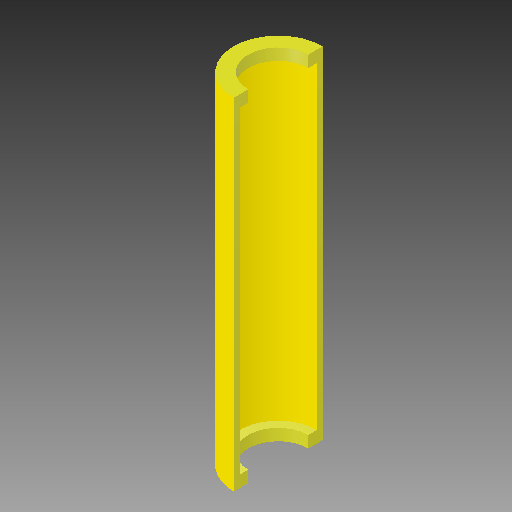
# Autodesk Inventor part: 蓋子
Saved by Autodesk Inventor 2017 (Build 210142000, 142)
## iProperties
Created: 2019-12-03
Part Number: 蓋子
Material: 一般
Document SubType Name: Modeling
Designer: 吳昇峻
Density: 1 g/cm^3
Appearance: 預設
Mass: 4.83432 g
Surface Area: 65.4473 cm^2
Volume: 4.83432 cm^3
Author: 吳昇峻
Autodesk Inventor part; units mm, degrees
ref_plane "YZ Plane" through (0, 0, 0) normal (1, 0, 0) x (0, 1, 0)
ref_plane "XZ Plane" through (0, 0, 0) normal (0, 1, 0) x (-1, 0, 0)
ref_plane "XY Plane" through (0, 0, 0) normal (0, 0, 1) x (1, 0, 0)
sketch "草圖1" plane through (0, 0, 0) normal (0, 1, 0) x (-1, 0, 0)
  arc A0 (0, -10) -> (0, 10) centre (0, 0) ccw
  arc A1 (0, -11.5) -> (0, 11.5) centre (0, 0) ccw
  line L0 (0, 11.5) -> (0, 10)
  line L1 (0, -10) -> (0, -11.5)
  dimension "d0" = 20
  dimension "d1" = 23
  constraints: 4 end point, 4 point on circle, 2 centre point, 2 coincident, 2 point on line, 1 vertical
  measures "d0" diameter of A0
  measures "d1" diameter of A1
extrude "擠出1" add sketch "草圖1" along normal blind 41
sketch "草圖2" plane through (0, 41, 0) normal (0, 1, 0) x (1, 0, 0)
  line L0 (0, -11.5) -> (0, -10) projected
  arc A0 (0, 11.5) -> (0, -11.5) centre (0, 0) ccw projected
  line L1 (0, 10) -> (0, 11.5) projected
  line L2 (0, -10) -> (0, 10)
  constraints: 2 end point, 1 vertical
extrude "擠出2" add sketch "草圖2" along normal blind 3
sketch "草圖3" plane through (0, 44, 0) normal (0, 1, 0) x (1, 0, 0)
  arc A0 (0, 7.75) -> (0, -7.75) centre (0, 0) ccw
  line L0 (0, -10) -> (0, 10) projected
  line L1 (0, -7.75) -> (0, 7.75)
  dimension "d7" = 15.5
  constraints: 2 end point, 2 point on circle, 2 point on line, 1 centre point, 1 coincident
  measures "d7" diameter of A0
extrude "擠出3" cut sketch "草圖3" against normal up to next
sketch "草圖5" plane through (0, 0, 0) normal (0, -1, 0) x (1, 0, 0)
  arc A0 (0, 10) -> (0, -10) centre (0, 0) ccw projected
  line L0 (0, 10) -> (0, 11.5) projected
  arc A1 (0, 11.5) -> (0, -11.5) centre (0, 0) ccw projected
  line L1 (0, -11.5) -> (0, -10) projected
  line L2 (0, 11.5) -> (0, -11.5)
  constraints: 2 end point, 1 vertical
extrude "擠出4" add sketch "草圖5" along normal blind 3
sketch "草圖7" plane through (0, -3, 0) normal (0, -1, 0) x (1, 0, 0)
  arc A0 (0, 7.75) -> (0, -7.75) centre (0, 0) ccw
  line L0 (0, -11.5) -> (0, 11.5) projected
  line L1 (0, -7.75) -> (0, 7.75)
  dimension "d13" = 15.5
  constraints: 2 end point, 2 point on circle, 2 point on line, 1 centre point, 1 coincident
  measures "d13" diameter of A0
extrude "擠出5" cut sketch "草圖7" against normal up to next
sketch "草圖8" plane through (0, 44, 0) normal (0, 1, 0) x (1, 0, 0)
  arc A0 (0, 11.5) -> (0, -11.5) centre (0, 0) ccw projected
  arc A1 (0, 10) -> (0, -10) centre (0, 0) ccw projected
  line L0 (0, 7.75) -> (0, 11.5) projected
  line L1 (0, 11.5) -> (0, 10)
  line L2 (0, -10) -> (0, -11.5)
  constraints: 4 end point, 2 collinear
extrude "擠出6" add sketch "草圖8" along normal blind 38
sketch "草圖9" plane through (0, 82, 0) normal (0, 1, 0) x (1, 0, 0)
  arc A0 (0, 11.5) -> (0, -11.5) centre (0, 0) ccw projected
  arc A1 (0, 7.75) -> (0, -7.75) centre (0, 0) ccw projected
  line L0 (0, 11.5) -> (0, 7.75) projected
  line L1 (0, -7.75) -> (0, -11.5) projected
extrude "擠出7" add sketch "草圖9" along normal blind 3
sketch "草圖10" plane through (0, 44, 0) normal (0, 1, 0) x (1, 0, 0)
  arc A0 (0, 10) -> (0, -10) centre (0, 0) ccw projected
  line L0 (0, -10) -> (0, -7.75) projected
  arc A1 (0, 7.75) -> (0, -7.75) centre (0, 0) ccw projected
  line L1 (0, 7.75) -> (0, 10) projected
extrude "擠出8" cut sketch "草圖10" against normal blind 3
sketch "Sketch11" plane through (0, 0, 0) normal (0, 0, 1) x (1, 0, 0)
  line L0 (0, 85) -> (-11.5, 85) projected
  line L1 (-11.5, -3) -> (0, -3) projected
  point P0 (0, 0)
  dimension "d22" = 88
  measures "d22" distance between parallel lines of L0 L1
